Barrel Mount Rotary Attachment_v10 (Autodesk Fusion 360 design; units mm, degrees)
Autodesk Fusion 360 part; units mm, degrees
note: some values were not read from the file. Set by a fixed rule: which sketch regions a step uses.
sketch "Sketch1" plane through (0, 0, 0) normal (1, 0, 0) x (0, 1, 0)
  line L0 (4.7917, 9.9987) -> (4.7522, 9.9948) construction
  line L1 (9.9948, 4.7522) -> (9.9987, 4.7917) construction
  line L2 (2.8393, 3.9) -> (0.207, 3.9) construction
  line L3 (9.8222, 4.4022) -> (9.8494, 4.4312) construction
  line L4 (9.8746, 4.4619) -> (9.8977, 4.4942) construction
  arc A0 (10, 9.5) -> (9.5, 10) centre (9.5, 9.5) ccw construction
  line L5 (4.8314, 10) -> (4.7917, 9.9987) construction
  line L6 (4.5279, 9.9187) -> (4.4942, 9.8977) construction
  line L7 (4.4942, 9.8977) -> (4.4619, 9.8746) construction
  line L8 (4.6363, 9.9678) -> (4.5991, 9.9538) construction
  line L9 (4.713, 9.9883) -> (4.6743, 9.9793) construction
  line L10 (0, 3.6952) -> (-0.2048, 3.9) construction
  line L11 (6.5607, 5.5) -> (8.2, 5.5) construction
  line L12 (10, 8.5) -> (10, 9.5) construction
  line L13 (4.563, 9.9374) -> (4.5279, 9.9187) construction
  line L14 (4.6743, 9.9793) -> (4.6363, 9.9678) construction
  line L15 (9.9987, 4.7917) -> (10, 4.9) construction
  line L16 (9.8977, 4.4942) -> (9.9187, 4.5279) construction
  line L17 (9.9187, 4.5279) -> (9.9374, 4.563) construction
  line L18 (10, 4.9) -> (10, 8.5) construction
  line L19 (4.4619, 9.8746) -> (4.4312, 9.8494) construction
  line L20 (4.7522, 9.9948) -> (4.713, 9.9883) construction
  line L21 (4.5991, 9.9538) -> (4.563, 9.9374) construction
  arc A1 (8.2, 3.2628) -> (8.5414, 3.1214) centre (8.4, 3.2628) ccw construction
  line L22 (0.207, 3.9) -> (0, 3.6952) construction
  line L23 (8.2, 5.5) -> (8.2, 3.2628) construction
  line L24 (9.8494, 4.4312) -> (9.8746, 4.4619) construction
  line L25 (-6.5607, 5.5) -> (-3.9, 2.8393) construction
  line L26 (-6.5607, 5.5) -> (-3.9, 2.8393) construction
  line L27 (-9.8977, 4.4942) -> (-9.8746, 4.4619) construction
  line L28 (-3.9, 0.1999) -> (-3.7001, 0) construction
  line L29 (-8.2, 5.5) -> (-6.5607, 5.5) construction
  line L30 (-9.9187, 4.5279) -> (-9.8977, 4.4942) construction
  line L31 (9.9374, 4.563) -> (9.9538, 4.5991) construction
  line L32 (9.9538, 4.5991) -> (9.9678, 4.6363) construction
  line L33 (9.9883, 4.713) -> (9.9948, 4.7522) construction
  line L34 (9.9678, 4.6363) -> (9.9793, 4.6743) construction
  line L35 (9.9793, 4.6743) -> (9.9883, 4.713) construction
  line L36 (-4.7522, 9.9948) -> (-4.7917, 9.9987) construction
  line L37 (-4.4619, 9.8746) -> (-4.4942, 9.8977) construction
  arc A2 (-3.2628, 8.2) -> (-3.1214, 8.5414) centre (-3.2628, 8.4) ccw construction
  line L38 (-10, 4.8314) -> (-9.9987, 4.7917) construction
  line L39 (-2.8393, 3.9) -> (-5.5, 6.5607) construction
  line L40 (-9.9987, 4.7917) -> (-9.9948, 4.7522) construction
  line L41 (-8.2, 3.2628) -> (-8.2, 5.5) construction
  line L42 (-10, 8.5) -> (-10, 4.8314) construction
  line L43 (-4.6743, 9.9793) -> (-4.713, 9.9883) construction
  line L44 (-4.4312, 9.8494) -> (-4.4619, 9.8746) construction
  line L45 (-3.9, 2.8393) -> (-3.9, 0.1999) construction
  line L46 (-9.8746, 4.4619) -> (-9.8494, 4.4312) construction
  line L47 (-9.9374, 4.563) -> (-9.9187, 4.5279) construction
  line L48 (-9.9793, 4.6743) -> (-9.9678, 4.6363) construction
  line L49 (-9.9987, 4.7917) -> (-9.9948, 4.7522) construction
  line L50 (-9.9678, 4.6363) -> (-9.9538, 4.5991) construction
  line L51 (-9.9538, 4.5991) -> (-9.9374, 4.563) construction
  line L52 (4.6363, 9.9678) -> (4.5991, 9.9538) construction
  line L53 (9.9678, 4.6363) -> (9.9793, 4.6743) construction
  line L54 (9.8746, 4.4619) -> (9.8977, 4.4942) construction
  line L55 (5.5, 8.2) -> (5.5, 6.5607) construction
  line L56 (-4.7522, 9.9948) -> (-4.7917, 9.9987) construction
  line L57 (-4.5991, 9.9538) -> (-4.6363, 9.9678) construction
  line L58 (-4.6363, 9.9678) -> (-4.6743, 9.9793) construction
  line L59 (4.5279, 9.9187) -> (4.4942, 9.8977) construction
  line L60 (-4.713, 9.9883) -> (-4.7522, 9.9948) construction
  line L61 (4.5991, 9.9538) -> (4.563, 9.9374) construction
  line L62 (0, 3.6952) -> (-0.2048, 3.9) construction
  line L63 (-4.5279, 9.9187) -> (-4.563, 9.9374) construction
  arc A3 (8.2, 3.2628) -> (8.5414, 3.1214) centre (8.4, 3.2628) ccw construction
  line L64 (9.9538, 4.5991) -> (9.9678, 4.6363) construction
  line L65 (-4.6743, 9.9793) -> (-4.713, 9.9883) construction
  line L66 (-4.563, 9.9374) -> (-4.5991, 9.9538) construction
  line L67 (4.4619, 9.8746) -> (4.4312, 9.8494) construction
  line L68 (-4.4942, 9.8977) -> (-4.5279, 9.9187) construction
  line L69 (10, 4.9) -> (10, 8.5) construction
  line L70 (9.9187, 4.5279) -> (9.9374, 4.563) construction
  line L71 (0.207, 3.9) -> (0, 3.6952) construction
  line L72 (3.9, -0.1999) -> (3.7001, 0) construction
  line L73 (2.8393, 3.9) -> (0.207, 3.9) construction
  arc A4 (-3.2628, 8.2) -> (-3.1214, 8.5414) centre (-3.2628, 8.4) ccw construction
  line L74 (-4.7917, 9.9987) -> (-4.8314, 10) construction
  line L75 (9.8977, 4.4942) -> (9.9187, 4.5279) construction
  line L76 (3.9, 0.1999) -> (3.9, 2.8393) construction
  line L77 (3.7001, 0) -> (3.9, 0.1999) construction
  line L78 (-9.9793, 4.6743) -> (-9.9678, 4.6363) construction
  line L79 (-4.4022, 9.8222) -> (-4.4312, 9.8494) construction
  line L80 (-9.9678, 4.6363) -> (-9.9538, 4.5991) construction
  line L81 (-5.5, 8.2) -> (-3.2628, 8.2) construction
  line L82 (-4.713, 9.9883) -> (-4.7522, 9.9948) construction
  line L83 (-4.5279, 9.9187) -> (-4.563, 9.9374) construction
  line L84 (-9.9538, 4.5991) -> (-9.9374, 4.563) construction
  line L85 (-4.8314, 10) -> (-8.5, 10) construction
  line L86 (-9.9883, 4.713) -> (-9.9793, 4.6743) construction
  line L87 (-4.6363, 9.9678) -> (-4.6743, 9.9793) construction
  line L88 (-9.9948, 4.7522) -> (-9.9883, 4.713) construction
  line L89 (-5.5, 6.5607) -> (-5.5, 8.2) construction
  line L90 (-4.7917, 9.9987) -> (-4.8314, 10) construction
  line L91 (-3.1214, 8.5414) -> (-4.4022, 9.8222) construction
  line L92 (4.4022, 9.8222) -> (3.1214, 8.5414) construction
  line L93 (9.5, 10) -> (4.8314, 10) construction
  line L94 (8.2, 5.5) -> (8.2, 3.2628) construction
  line L95 (8.5414, 3.1214) -> (9.8222, 4.4022) construction
  line L96 (4.4312, 9.8494) -> (4.4022, 9.8222) construction
  line L97 (8.5414, 3.1214) -> (9.8222, 4.4022) construction
  line L98 (5.5, 6.5607) -> (2.8393, 3.9) construction
  line L99 (3.2628, 8.2) -> (5.5, 8.2) construction
  arc A5 (3.1214, 8.5414) -> (3.2628, 8.2) centre (3.2628, 8.4) ccw construction
  line L100 (-2.8393, 3.9) -> (-5.5, 6.5607) construction
  line L101 (5.5, 6.5607) -> (2.8393, 3.9) construction
  line L102 (-10, 8.5) -> (-10, 4.8314) construction
  line L103 (3.9, -0.1999) -> (3.7001, 0) construction
  line L104 (3.7001, 0) -> (3.9, 0.1999) construction
  line L105 (3.9, 2.8393) -> (6.5607, 5.5) construction
  line L106 (5.5, 8.2) -> (5.5, 6.5607) construction
  line L107 (-5.5, 6.5607) -> (-5.5, 8.2) construction
  line L108 (3.9, 2.8393) -> (6.5607, 5.5) construction
  line L109 (-0.2048, 3.9) -> (-2.8393, 3.9) construction
  line L110 (3.9, 0.1999) -> (3.9, 2.8393) construction
  line L111 (-5.5, 8.2) -> (-3.2628, 8.2) construction
  line L112 (-4.8314, 10) -> (-8.5, 10) construction
  line L113 (-9.8494, 4.4312) -> (-9.8222, 4.4022) construction
  line L114 (-9.8977, 4.4942) -> (-9.8746, 4.4619) construction
  line L115 (-10, 9.5) -> (-10, 8.5) construction
  line L116 (-9.9883, 4.713) -> (-9.9793, 4.6743) construction
  arc A6 (-9.5, 10) -> (-10, 9.5) centre (-9.5, 9.5) ccw construction
  line L117 (-8.5, 10) -> (-9.5, 10) construction
  line L118 (-9.9187, 4.5279) -> (-9.8977, 4.4942) construction
  line L119 (-4.5991, 9.9538) -> (-4.6363, 9.9678) construction
  line L120 (-9.9374, 4.563) -> (-9.9187, 4.5279) construction
  line L121 (-4.4942, 9.8977) -> (-4.5279, 9.9187) construction
  line L122 (-9.8746, 4.4619) -> (-9.8494, 4.4312) construction
  line L123 (-4.563, 9.9374) -> (-4.5991, 9.9538) construction
  line L124 (-8.2, 3.2628) -> (-8.2, 5.5) construction
  arc A7 (-8.5414, 3.1214) -> (-8.2, 3.2628) centre (-8.4, 3.2628) ccw construction
  line L125 (-9.8222, 4.4022) -> (-8.5414, 3.1214) construction
  line L126 (4.563, 9.9374) -> (4.5279, 9.9187) construction
  line L127 (-3.1214, 8.5414) -> (-4.4022, 9.8222) construction
  line L128 (9.9793, 4.6743) -> (9.9883, 4.713) construction
  line L129 (9.9374, 4.563) -> (9.9538, 4.5991) construction
  line L130 (9.5, 10) -> (4.8314, 10) construction
  line L131 (4.6743, 9.9793) -> (4.6363, 9.9678) construction
  line L132 (10, 8.5) -> (10, 9.5) construction
  line L133 (4.7522, 9.9948) -> (4.713, 9.9883) construction
  line L134 (3.2628, 8.2) -> (5.5, 8.2) construction
  arc A8 (10, 9.5) -> (9.5, 10) centre (9.5, 9.5) ccw construction
  line L135 (-8.5, 10) -> (-9.5, 10) construction
  line L136 (4.713, 9.9883) -> (4.6743, 9.9793) construction
  line L137 (4.7917, 9.9987) -> (4.7522, 9.9948) construction
  line L138 (9.9948, 4.7522) -> (9.9987, 4.7917) construction
  line L139 (-4.4312, 9.8494) -> (-4.4619, 9.8746) construction
  line L140 (-10, 9.5) -> (-10, 8.5) construction
  line L141 (-4.4022, 9.8222) -> (-4.4312, 9.8494) construction
  line L142 (9.8222, 4.4022) -> (9.8494, 4.4312) construction
  arc A9 (-9.5, 10) -> (-10, 9.5) centre (-9.5, 9.5) ccw construction
  line L143 (9.8494, 4.4312) -> (9.8746, 4.4619) construction
  line L144 (4.4022, 9.8222) -> (3.1214, 8.5414) construction
  line L145 (4.8314, 10) -> (4.7917, 9.9987) construction
  line L146 (9.9987, 4.7917) -> (10, 4.9) construction
  line L147 (4.4942, 9.8977) -> (4.4619, 9.8746) construction
  line L148 (-4.4619, 9.8746) -> (-4.4942, 9.8977) construction
  arc A10 (3.1214, 8.5414) -> (3.2628, 8.2) centre (3.2628, 8.4) ccw construction
  line L149 (4.4312, 9.8494) -> (4.4022, 9.8222) construction
  line L150 (9.9883, 4.713) -> (9.9948, 4.7522) construction
  line L151 (6.5607, 5.5) -> (8.2, 5.5) construction
  line L152 (-3.9, 0.1999) -> (-3.7001, 0) construction
  line L153 (-9.9948, 4.7522) -> (-9.9883, 4.713) construction
  line L154 (-9.8222, 4.4022) -> (-8.5414, 3.1214) construction
  line L155 (-3.7001, 0) -> (-3.9, -0.1999) construction
  line L156 (-3.7001, 0) -> (-3.9, -0.1999) construction
  line L157 (-8.2, 5.5) -> (-6.5607, 5.5) construction
  line L158 (-9.8494, 4.4312) -> (-9.8222, 4.4022) construction
  line L159 (-3.9, 2.8393) -> (-3.9, 0.1999) construction
  arc A11 (-8.5414, 3.1214) -> (-8.2, 3.2628) centre (-8.4, 3.2628) ccw construction
  line L160 (-0.2048, 3.9) -> (-2.8393, 3.9) construction
  line L161 (-10, 4.8314) -> (-9.9987, 4.7917) construction
  line L162 (-3.0507, 8.6121) -> (-4.3315, 9.8929)
  line L163 (4.3315, 9.8929) -> (3.0507, 8.6121)
  line L164 (-4.8314, 10.1) -> (-3.6911, 10.1) construction
  line L165 (-4.8314, 10.1) -> (-4.5386, 10.1) construction
  line L166 (-4.3315, 9.8929) -> (-4.5386, 10.1)
  line L167 (4.8314, 10.1) -> (4.5386, 10.1) construction
  line L168 (4.3315, 9.8929) -> (4.5386, 10.1)
  line L169 (4.5386, 10.1) -> (14.5386, 10.1)
  line L170 (-4.5386, 10.1) -> (-14.5386, 10.1)
  line L171 (-3.0507, 8.6121) -> (3.0507, 8.6121)
  line L172 (-14.5386, 10.1) -> (-14.5386, 17.1)
  line L173 (14.5386, 10.1) -> (14.5386, 17.1)
  line L174 (-14.5386, 17.1) -> (14.5386, 17.1)
  dimension "d1" = 0.1
  dimension "d2" = 0.1
  dimension "d5" = 10
  dimension "d6" = 10
  dimension "d7" = 7
  dimension "d8" = 7
  constraint coincident L164 L165.end
  constraint parallel L130 L169
  constraint parallel L112 L170
  constraint horizontal L171
  constraint coincident L163 L171.end
  constraint perpendicular L170 L172
  constraint perpendicular L169 L173
  measures "d5" distance of L167.end L169.end
  measures "d6" distance of L165.end L170.end
  measures "d7" distance of L170.end L172.end
  measures "d8" distance of L169.end L173.end
  measures "d16" diameter of L3.start
  measures "d17" diameter of L3.start
extrude "Extrude1" add sketch "Sketch1" along normal blind 45
sketch "Sketch2" plane through (0, 0, 17.1) normal (0, 0, 1) x (-1, 0, 0)
  line L0 (0, -14.5386) -> (0, 14.5386)
  line L1 (0, 14.5386) -> (-45, 14.5386)
  line L2 (-45, 14.5386) -> (-45, -14.5386)
  line L3 (-45, -14.5386) -> (0, -14.5386)
  circle A0 centre (-22.5, 0) radius 2.5
  circle A1 centre (-8, 0) radius 2.7
  circle A2 centre (-37, 0) radius 2.7
  line L4 (-19.7, -6.9443) -> (-25.3, -6.9443)
  line L5 (-25.3, -6.9443) -> (-25.3, -5.0443)
  line L6 (-25.3, -5.0443) -> (-19.7, -5.0443)
  line L7 (-19.7, -5.0443) -> (-19.7, -6.9443)
  line L8 (-19.7, -6.9443) -> (-25.3, -5.0443) construction
  line L9 (-25.3, -6.9443) -> (-19.7, -5.0443) construction
  line L10 (-22.5, -14.5386) -> (-22.5, 14.5386) construction
  line L11 (0, -5.9943) -> (-45, -5.9943) construction
  circle A3 centre (-22.5, 0) radius 27.425 construction
  line L12 (-22.5, 0) -> (-14.2578, 0) construction
  line L13 (-19.7, 6.9443) -> (-25.3, 6.9443)
  line L14 (-19.7, 5.0443) -> (-19.7, 6.9443)
  line L15 (-25.3, 5.0443) -> (-19.7, 5.0443)
  line L16 (-25.3, 6.9443) -> (-25.3, 5.0443)
  point P0 (-22.5, -5.9943)
  dimension "d11" = 5
  dimension "d12" = 5.4
  dimension "d13" = 5.4
  dimension "d22" = 5.6
  dimension "d23" = 1.9
  dimension "d26" = 54.85
  constraint horizontal L4
  constraint perpendicular L4 L5
  constraint parallel L4 L6
  constraint parallel L5 L7
  constraint coincident L8 P0
  constraint coincident L9 P0
  constraint midpoint L3 L10.start
  constraint midpoint L1 L10.end
  constraint coincident P0 L10
  constraint midpoint A0.centre L10
  constraint coincident L0 L11.start
  constraint coincident L2 L11.end
  constraint perpendicular L2 L11
  constraint midpoint P0 L11
  constraint concentric A0 A3
  constraint coincident A0.centre A3.centre
  constraint perpendicular L10 L12
  constraint symmetric L4.start L12 L13.start
  constraint symmetric L4.end L12 L13.end
  constraint symmetric L5.end L12 L15.start
  constraint symmetric L6.end L12 L14.start
  measures "d11" diameter of A0
  measures "d12" diameter of A1
  measures "d13" diameter of A2
  measures "d22" distance of L5.end L6.end
  measures "d23" distance of L4.end L5.end
  measures "d26" diameter of A3
extrude "Extrude2" cut sketch "Sketch2" against normal blind 8.5 contours A0 | A1 | A2
sketch "Sketch3" plane through (0, 14.5386, 0) normal (0, 1, 0) x (-1, 0, 0)
  line L0 (0, 10.1) -> (0, 17.1)
  line L1 (0, 17.1) -> (-45, 17.1)
  line L2 (-45, 17.1) -> (-45, 10.1)
  line L3 (-45, 10.1) -> (0, 10.1)
  circle A0 centre (-22.5, 13.6) radius 1.55
  circle A1 centre (-22.5, 13.6) radius 3
  line L4 (-45, 17.1) -> (0, 10.1) construction
  line L5 (0, 17.1) -> (-45, 10.1) construction
  dimension "d16" = 3.1
  dimension "d17" = 6
  constraint concentric A0 A1
  constraint coincident L1.end L2.start
  constraint coincident L0.start L3.end
  constraint coincident L0.end L1.start
  constraint coincident L2.end L3.start
  constraint midpoint A0.centre L5
  measures "d16" diameter of A0
  measures "d17" diameter of A1
extrude "Extrude3" cut sketch "Sketch3" against normal blind 2 contours A1
extrude "Extrude4" cut sketch "Sketch3" against normal blind 15 contours A0
extrude "Extrude5" cut sketch "Sketch2" against normal blind 6.5 contours L4 L5 L6 L7
extrude "Extrude6" cut sketch "Sketch2" against normal blind 6.5 contours L13 L14 L15 L16
sketch "Sketch4" plane through (0, -14.5386, 0) normal (0, -1, 0) x (1, 0, 0)
  line L0 (0, 17.1) -> (0, 10.1)
  line L1 (0, 10.1) -> (45, 10.1)
  line L2 (45, 10.1) -> (45, 17.1)
  line L3 (45, 17.1) -> (0, 17.1)
  line L4 (0, 17.1) -> (45, 10.1) construction
  line L5 (45, 17.1) -> (0, 10.1) construction
  circle A0 centre (22.5, 13.6) radius 1.55
  circle A1 centre (22.5, 13.6) radius 3
  dimension "d29" = 3.1
  dimension "d30" = 6
  constraint coincident L0.start L3.end
  constraint coincident L1.end L2.start
  constraint coincident L2.end L3.start
  constraint coincident L0.end L1.start
  constraint midpoint L5 A0.centre
  constraint concentric A0 A1
  measures "d29" diameter of A0
  measures "d30" diameter of A1
extrude "Extrude7" cut sketch "Sketch4" against normal blind 15 contours A0
extrude "Extrude8" cut sketch "Sketch4" against normal blind 2 contours A1
